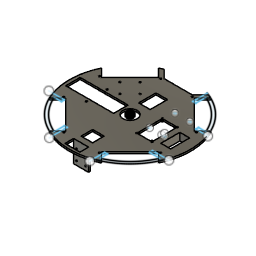
全国ディフェンス上面v3 v4 (Autodesk Fusion 360 design; units mm, degrees)
Autodesk Fusion 360 part; units mm, degrees
note: some values were not read from the file. Set by a fixed rule: which sketch regions a step uses.
sketch "スケッチ1" plane through (0, 0, 0) normal (0, 0, 1) x (1, 0, 0)
sketch "スケッチ2" plane through (0, 0, 0) normal (0, 0, 1) x (1, 0, 0)
  line L0 (105, 0) -> (105, 35)
  line L1 (105, 35) -> (98.9949, 35)
  line L2 (98.9949, 35) -> (78.9949, 35)
  line L3 (78.9949, 35) -> (105, 35)
  line L4 (105, 35) -> (105, -35)
  line L5 (105, -35) -> (78.9949, -35)
  line L6 (78.9949, -35) -> (78.9949, 35)
  line L7 (0, 105) -> (35, 105)
  line L8 (35, 105) -> (-35, 105)
  line L9 (-35, 105) -> (-35, 78.995)
  line L10 (-35, 78.995) -> (35, 78.995)
  line L11 (35, 78.995) -> (35, 105)
  line L12 (-105, 0) -> (-105, -35)
  line L13 (-105, -35) -> (-78.995, -35)
  line L14 (-78.995, -35) -> (-78.995, 34.9927)
  line L15 (-78.995, 34.9927) -> (-105, 34.9927)
  line L16 (-105, 34.9927) -> (-105, -35)
  line L17 (0, -105) -> (35, -105)
  line L18 (35, -105) -> (-35, -105)
  line L19 (-35, -105) -> (-35, -78.995)
  line L20 (-35, -78.995) -> (35, -78.995)
  line L21 (35, -78.995) -> (35, -105)
  arc A0 (-98.9949, -35) -> (-35, -98.9949) centre (0, 0) ccw
  arc A1 (35, -98.9949) -> (98.9949, -35) centre (0, 0) ccw
  arc A2 (98.9949, 35) -> (35, 98.9949) centre (0, 0) ccw
  arc A3 (-35, 98.9949) -> (-98.9975, 34.9927) centre (0, 0) ccw
  line L22 (-35, 98.9949) -> (-42, 98.9949)
  line L23 (-42, 98.9949) -> (-42, 96.2341)
  line L24 (-42, 96.2341) -> (-42, 76.2341)
  line L25 (-98.9975, 34.9927) -> (-98.9975, 42)
  line L26 (-98.9975, 42) -> (-96.2341, 42)
  line L27 (-96.2341, 42) -> (-76.2341, 42)
  line L28 (-76.2341, 42) -> (-42, 76.2341)
  dimension "d2" = 35
  dimension "d3" = 20
  dimension "d4" = 70
  dimension "d5" = 26.005
  dimension "d6" = 26.005
  dimension "d7" = 70
  dimension "d8" = 26.005
  dimension "d9" = 20
  dimension "d10" = 20
  constraint vertical L0
  constraint perpendicular L0 L1
  constraint perpendicular L0 L2
  constraint horizontal L3
  constraint vertical L4
  constraint horizontal L5
  constraint vertical L6
  constraint horizontal L7
  constraint horizontal L8
  constraint vertical L9
  constraint horizontal L10
  constraint vertical L11
  constraint vertical L12
  constraint horizontal L13
  constraint vertical L14
  constraint horizontal L15
  constraint vertical L16
  constraint horizontal L17
  constraint horizontal L18
  constraint vertical L19
  constraint horizontal L20
  constraint vertical L21
  constraint coincident L13 A0.start
  constraint coincident L19 A0.end
  constraint coincident L5 A1.end
  constraint coincident L21 A1.start
  constraint coincident L11 A2.end
  constraint coincident A0.centre A1.centre
  constraint coincident L15 A3.end
  constraint coincident L9 A3.start
  constraint perpendicular L9 L22
  constraint coincident A3 L23.end
  constraint perpendicular L22 L23
  constraint perpendicular L22 L24
  constraint perpendicular L15 L25
  constraint coincident A3 L26.end
  constraint perpendicular L25 L26
  constraint parallel L26 L27
  measures "d2" distance of L0.start L0.end
  measures "d3" distance of L1.end L2.end
  measures "d4" distance of L7.end L8.end
  measures "d5" distance of L7.end L10.end
  measures "d6" distance of L12.end L13.end
  measures "d7" distance of L17.end L18.end
  measures "d8" distance of L17.end L20.end
  measures "d9" distance of L23.end L24.end
  measures "d10" distance of L26.end L27.end
sketch "スケッチ3" plane through (0, 0, 0) normal (0, 0, 1) x (1, 0, 0)
  line L0 (-79, 35) -> (-74, 35)
  line L1 (-76.5, 35) -> (-76.5, 37.5)
  line L2 (-35, 79) -> (-35, 74)
  line L3 (-35, 74) -> (-35, 75)
  line L4 (-35, 76.5) -> (-37.5, 76.5)
  circle A0 centre (-37.5, 76.5) radius 1.5
  circle A1 centre (-76.5, 37.5) radius 1.5
  dimension "d11" = 3
  dimension "d12" = 3
  constraint horizontal L0
  constraint midpoint L0 L1.start
  constraint perpendicular L0 L1
  constraint vertical L2
  constraint coincident L2 L3.end
  constraint midpoint L2 L4.start
  constraint perpendicular L2 L4
  constraint coincident L4.end A0.centre
  constraint coincident L1.end A1.centre
  measures "d11" diameter of A0
  measures "d12" diameter of A1
extrude "押し出し1" add sketch "スケッチ2" along normal blind 3 contours L2 L3 L5 L6 L9 L10 L11 L13 L14 L15 L19 L20 L21 A0 A1 A2 A3 L24 L27 L28
extrude "押し出し2" cut sketch "スケッチ3" along normal blind 3
sketch "スケッチ4" plane through (0, 0, 0) normal (0, 0, 1) x (1, 0, 0)
sketch "スケッチ5" plane through (0, 0, 3) normal (0, 0, 1) x (-1, 0, 0)
  circle A0 centre (76.5, -37.5) radius 1.5
  circle A1 centre (37.5, -76.5) radius 1.5
  arc A2 (96.2341, -42) -> (98.9975, -34.9927) centre (0, 0) ccw
  line L0 (98.9975, -34.9927) -> (78.995, -34.9927)
  line L1 (78.995, -34.9927) -> (78.995, 35)
  line L2 (78.995, 35) -> (98.9949, 35)
  arc A3 (98.9949, 35) -> (35, 98.9949) centre (0, 0) ccw
  line L3 (35, 98.9949) -> (35, 78.995)
  line L4 (35, 78.995) -> (-35, 78.995)
  line L5 (-35, 78.995) -> (-35, 98.9949)
  arc A4 (-35, 98.9949) -> (-98.9949, 35) centre (0, 0) ccw
  line L6 (-98.9949, 35) -> (-78.9949, 35)
  line L7 (-78.9949, 35) -> (-78.9949, -35)
  line L8 (-78.9949, -35) -> (-98.9949, -35)
  arc A5 (-98.9949, -35) -> (-35, -98.9949) centre (0, 0) ccw
  line L9 (-35, -98.9949) -> (-35, -78.995)
  line L10 (-35, -78.995) -> (35, -78.995)
  line L11 (35, -78.995) -> (35, -98.9949)
  arc A6 (35, -98.9949) -> (42, -96.2341) centre (0, 0) ccw
  line L12 (42, -96.2341) -> (42, -76.2341)
  line L13 (42, -76.2341) -> (76.2341, -42)
  line L14 (76.2341, -42) -> (96.2341, -42)
  line L15 (78.995, -34.9927) -> (78.995, -40)
  line L16 (78.995, -40) -> (74, -40)
  line L17 (35, -78.995) -> (40, -78.995)
  line L18 (40, -78.995) -> (40, -74)
  line L19 (40, -74) -> (74, -40)
  constraint coincident L0.end L1.start
  constraint perpendicular L0 L15
  constraint perpendicular L15 L16
  constraint coincident L10.end L11.start
  constraint perpendicular L11 L17
  constraint perpendicular L10 L18
sketch "スケッチ6" plane through (0, 0, 3) normal (0, 0, 1) x (-1, 0, 0)
  line L0 (-35, -79) -> (-35, -74)
  line L1 (-35, -74) -> (-40, -74)
  arc A0 (-91.6515, -40) -> (-40, -91.6515) centre (0, 0) ccw
  line L2 (-79, -35) -> (-100, -35)
  line L3 (-79, -35) -> (-79, -40)
  arc A1 (-98.9949, -35) -> (-34.9984, -98.9955) centre (0, 0) ccw
  line L4 (-34.9984, -98.9955) -> (-35, -79)
  line L5 (-40, -74) -> (-40, -91.6515)
  line L6 (-91.6515, -40) -> (-79, -40)
  line L7 (-79, 35) -> (-74, 35)
  line L8 (-74, 35) -> (-74, 40)
  line L9 (-79, 35) -> (-102.5239, 35)
  line L10 (-35, 79) -> (-40, 79)
  line L11 (-35, 79) -> (-35, 105)
  arc A2 (-35, 98.9949) -> (-98.9949, 35) centre (0, 0) ccw
  arc A3 (-40, 91.6515) -> (-91.6515, 40) centre (0, 0) ccw
  line L12 (-40, 79) -> (-40, 91.6515)
  line L13 (-74, 40) -> (-91.6515, 40)
  line L14 (35, 79) -> (35, 74)
  line L15 (35, 74) -> (40, 74)
  line L16 (35, 79) -> (35, 105)
  line L17 (79, 35) -> (79, 40)
  line L18 (79, 35) -> (106, 35)
  arc A4 (98.9949, 35) -> (35, 98.9949) centre (0, 0) ccw
  arc A5 (91.6515, 40) -> (40, 91.6515) centre (0, 0) ccw
  line L19 (91.6515, 40) -> (79, 40)
  line L20 (40, 74) -> (40, 91.6515)
  dimension "d17" = 100
  dimension "d18" = 105
  dimension "d19" = 105
  dimension "d20" = 100
  dimension "d21" = 105
  dimension "d22" = 100
  constraint vertical L0
  constraint perpendicular L0 L1
  constraint coincident A0.centre A1.centre
  constraint perpendicular L2 L3
  constraint coincident L2 A1.start
  constraint perpendicular L1 L5
  constraint perpendicular L3 L6
  constraint horizontal L7
  constraint perpendicular L7 L8
  constraint parallel L7 L9
  constraint horizontal L10
  constraint perpendicular L10 L11
  constraint coincident L11 A2.start
  constraint coincident L9 A2.end
  constraint perpendicular L10 L12
  constraint perpendicular L8 L13
  constraint vertical L14
  constraint perpendicular L14 L15
  constraint parallel L14 L16
  constraint vertical L17
  constraint perpendicular L17 L18
  constraint coincident L18 A4.start
  constraint coincident L16 A4.end
  constraint perpendicular L17 L19
  constraint perpendicular L15 L20
  measures "d17" radius of A0
  measures "d18" radius of A1
  measures "d19" radius of A2
  measures "d20" radius of A3
  measures "d21" radius of A4
  measures "d22" radius of A5
sketch "スケッチ7" plane through (0, 0, 3) normal (0, 0, 1) x (-1, 0, 0)
  line L0 (79, 35) -> (74, 35)
  line L1 (76.5, 35) -> (76.5, 37.5)
  line L2 (37.5, 74) -> (37.5, 76.5)
  line L3 (-37.5, 79) -> (-37.5, 76.5)
  line L4 (-74, 37.5) -> (-76.5, 37.5)
  circle A0 centre (-76.5, -37.5) radius 1.5
  circle A1 centre (-37.5, -76.5) radius 1.5
  circle A2 centre (-76.5, 37.5) radius 1.5
  circle A3 centre (-37.5, 76.5) radius 1.5
  circle A4 centre (37.5, 76.5) radius 1.5
  circle A5 centre (76.5, 37.5) radius 1.5
  dimension "d23" = 2.5
  dimension "d24" = 3
  dimension "d25" = 3
  constraint horizontal L0
  constraint midpoint L0 L1.start
  constraint perpendicular L0 L1
  constraint vertical L2
  constraint vertical L3
  constraint horizontal L4
  constraint coincident L4.end A2.centre
  constraint coincident L3.end A3.centre
  constraint coincident L2.end A4.centre
  constraint coincident L1.end A5.centre
  measures "d23" distance of L1.start L1.end
  measures "d24" diameter of A2
  measures "d25" diameter of A5
extrude "押し出し3" cut sketch "スケッチ7" against normal blind 3
sketch "スケッチ8" plane through (0, 0, 3) normal (0, 0, 1) x (-1, 0, 0)
  line L0 (-68, 68) -> (-59.1612, 76.8388)
  line L1 (-68, 68) -> (-76.8388, 59.1612)
  line L2 (-76.8388, 59.1612) -> (-20.9774, 3.2997)
  line L3 (-20.9774, 3.2997) -> (-3.2997, 20.9774)
  line L4 (-3.2997, 20.9774) -> (-59.1612, 76.8388)
  line L5 (-76.8388, 59.1612) -> (-80.7279, 55.2721)
  line L6 (-80.7279, 55.2721) -> (-55.2721, 29.8162)
  line L7 (-55.2721, 29.8162) -> (-51.383, 33.7053)
  line L8 (-51.7365, 26.2807) -> (-47.8475, 30.1698)
  arc A0 (-55.2721, 29.8162) -> (-51.7365, 26.2807) centre (-53.5043, 28.0485) ccw
  circle A1 centre (-53.5043, 28.0485) radius 1.5
  line L9 (-53.5043, 28.0485) -> (-28.0485, 53.5043)
  circle A2 centre (-28.0485, 53.5043) radius 1.5
  dimension "d28" = 12.5
  dimension "d29" = 12.5
  dimension "d30" = 79
  dimension "d31" = 25
  dimension "d33" = 5.5
  dimension "d34" = 36
  dimension "d35" = 5
  dimension "d36" = 3
  dimension "d37" = 36
  dimension "d38" = 3
  constraint perpendicular L1 L2
  constraint perpendicular L2 L5
  constraint perpendicular L5 L6
  constraint coincident L2 L7.end
  constraint perpendicular L2 L7
  constraint coincident L2 L8.end
  constraint perpendicular L2 L8
  constraint concentric A0 A1
  constraint coincident A0.centre A1.centre
  constraint perpendicular L4 L9
  constraint coincident L9.end A2.centre
  measures "d28" distance of L0.start L0.end
  measures "d29" distance of L0.start L1.end
  measures "d30" distance of L1.end L2.end
  measures "d31" distance of L2.end L3.end
  measures "d33" distance of L1.end L5.end
  measures "d34" distance of L5.end L6.end
  measures "d35" distance of L6.end L8.start
  measures "d36" diameter of A1
  measures "d37" distance of A0.centre L9.end
  measures "d38" diameter of A2
extrude "押し出し4" cut sketch "スケッチ8" against normal blind 3 contours A1 | A2
sketch "スケッチ9" plane through (0, 0, 3) normal (0, 0, 1) x (-1, 0, 0)
  line L0 (-53.5, 28) -> (-81.4307, 55.9307)
  arc A0 (-55.2678, 29.7678) -> (-51.7322, 26.2322) centre (-53.5, 28) ccw
  line L1 (-55.2678, 29.7678) -> (-51.3787, 33.6569)
  line L2 (-81.4307, 55.9307) -> (-77.5416, 59.8198)
  line L3 (-77.5416, 59.8198) -> (-21.6802, 3.9584)
  line L4 (-21.6802, 3.9584) -> (-4.0025, 21.636)
  line L5 (-4.0025, 21.636) -> (-59.864, 77.4975)
  line L6 (-59.864, 77.4975) -> (-77.5416, 59.8198)
  dimension "d43" = 39.5
  dimension "d44" = 2.5
  dimension "d45" = 5.5
  dimension "d46" = 5.5
  dimension "d47" = 79
  dimension "d48" = 25
  dimension "d49" = 79
  constraint coincident L0.start A0.centre
  constraint perpendicular L0 L1
  constraint perpendicular L0 L2
  constraint perpendicular L1 L3
  constraint perpendicular L4 L5
  constraint perpendicular L3 L6
  measures "d43" distance of L0.start L0.end
  measures "d44" radius of A0
  measures "d45" distance of A0.start L1.end
  measures "d46" distance of L0.end L2.end
  measures "d47" distance of L2.end L3.end
  measures "d48" distance of L3.end L4.end
  measures "d49" distance of L4.end L5.end
extrude "押し出し5" cut sketch "スケッチ9" against normal blind 90 contours L3 L4 L5 L6
sketch "スケッチ10" plane through (0, 0, 3) normal (0, 0, 1) x (-1, 0, 0)
sketch "スケッチ11" plane through (0, 0, 0) normal (0, 0, 1) x (1, 0, 0)
sketch "スケッチ12" plane through (0, 0, 0) normal (0, 0, 1) x (1, 0, 0)
sketch "スケッチ13" plane through (0, 0, 0) normal (0, 0, 1) x (1, 0, 0)
sketch "スケッチ14" plane through (0, 0, 3) normal (0, 0, 1) x (-1, 0, 0)
  circle A0 centre (76.5, 37.5) radius 1.5
  circle A1 centre (37.5, 76.5) radius 1.5
  circle A2 centre (-37.5, 76.5) radius 1.5
  circle A3 centre (-76.5, 37.5) radius 1.5
  circle A4 centre (-76.5, -37.5) radius 1.5
  circle A5 centre (-37.5, -76.5) radius 1.5
  dimension "d71" = 3
  measures "d71" diameter of A0
extrude "押し出し6" add sketch "スケッチ14" against normal blind 3
sketch "スケッチ15" plane through (0, 0, 3) normal (0, 0, 1) x (-1, 0, 0)
extrude "押し出し7" add sketch "スケッチ5" along normal blind 3
move_face "面をオフセット1" offset -3 1 faces at (-50.128, -6.7155, 0)
sketch "スケッチ16" plane through (0, 0, 0) normal (0, 0, 1) x (1, 0, 0)
move_body "移動1" bodies 1 to x (0.707107, -0.707107, 0) y (0.707107, 0.707107, 0) z (0, 0, 1) at (-0.0004, -0.0009, -3)
sketch "スケッチ17" plane through (0, 0, 0) normal (0, 0, 1) x (1, 0, 0)
  line L0 (0, 0) -> (-16, 0)
  line L1 (-16, 0) -> (-16, 12.5)
  line L2 (-16, 12.5) -> (-99.104, 12.5)
  line L3 (-99.104, 12.5) -> (-99.104, -12.5)
  line L4 (-99.104, -12.5) -> (-16, -12.5)
  line L5 (-16, -12.5) -> (-16, 12.5)
  circle A0 centre (0, 0) radius 12.5
  line L6 (-57.552, 12.5) -> (-57.552, 0)
  line L7 (-57.552, 0) -> (-57.552, 18)
  line L8 (-57.552, 18) -> (-99.0603, 18)
  line L9 (-57.552, 18) -> (-57.552, -18)
  circle A1 centre (-57.552, 18) radius 1.5
  circle A2 centre (-57.552, -18) radius 1.5
  dimension "d77" = 16
  dimension "d78" = 12.5
  dimension "d79" = 83.104
  dimension "d80" = 25
  dimension "d81" = 25
  dimension "d82" = 18
  dimension "d84" = 3
  dimension "d85" = 3
  constraint coincident L0.start A0.centre
  constraint horizontal L0
  constraint perpendicular L0 L1
  constraint horizontal L2
  constraint vertical L3
  constraint horizontal L4
  constraint vertical L5
  constraint midpoint L2 L6.start
  constraint perpendicular L2 L6
  constraint perpendicular L2 L7
  constraint perpendicular L7 L8
  constraint perpendicular L4 L9
  constraint coincident L7.end L8.start
  constraint coincident L9.end A2.centre
  measures "d77" distance of L0.start L0.end
  measures "d78" distance of L0.end L1.end
  measures "d79" distance of L1.end L2.end
  measures "d80" distance of L1.end L4.end
  measures "d81" diameter of A0
  measures "d82" distance of L6.end L7.end
  measures "d84" diameter of A1
  measures "d85" diameter of A2
extrude "押し出し8" cut sketch "スケッチ17" along normal blind 3
sketch "スケッチ18" plane through (0, 0, 0) normal (0, 0, 1) x (1, 0, 0)
  circle A0 centre (60, 44) radius 1.5
  circle A1 centre (34, 44) radius 1.5
  circle A2 centre (60, 0) radius 1.5
  circle A3 centre (34, 0) radius 1.5
  line L0 (55, 0) -> (55, 5)
  dimension "d88" = 26
  dimension "d89" = 44
  dimension "d90" = 3
  dimension "d91" = 3
  dimension "d92" = 3
  dimension "d93" = 3
  measures "d88" distance of A2.centre A3.centre
  measures "d89" distance of A0.centre A2.centre
  measures "d90" diameter of A0
  measures "d91" diameter of A1
  measures "d92" diameter of A2
  measures "d93" diameter of A3
sketch "スケッチ19" plane through (0, 0, 0) normal (0, 0, -1) x (1, 0, 0)
  line L0 (-99.104, 12.5) -> (-16, 12.5)
  line L1 (-16, 12.5) -> (-16, -12.5)
  line L2 (-16, -12.5) -> (-99.104, -12.5)
  line L3 (-99.104, -12.5) -> (-99.104, 12.5)
  circle A0 centre (-57.552, -18) radius 1.5
  circle A1 centre (0, 0) radius 12.5
  circle A2 centre (-57.552, 18) radius 1.5
  circle A3 centre (-27.5775, -80.6093) radius 1.5
  circle A4 centre (27.5768, -80.6093) radius 1.5
  arc A5 (-45.2586, -94.7445) -> (-38.3497, -97.7454) centre (-0.0004, 0.0009) ccw
  line L4 (-38.3497, -97.7454) -> (-24.2075, -83.6032)
  line L5 (-24.2075, -83.6032) -> (24.2068, -83.6032)
  line L6 (24.2068, -83.6032) -> (38.3489, -97.7454)
  arc A6 (38.3489, -97.7454) -> (45.2509, -94.7478) centre (-0.0004, 0.0009) ccw
  line L7 (45.2509, -94.7478) -> (31.1088, -80.6057)
  line L8 (31.1088, -80.6057) -> (80.6063, -31.1083)
  line L9 (80.6063, -31.1083) -> (94.7484, -45.2504)
  arc A7 (94.7484, -45.2504) -> (94.7484, 45.2522) centre (-0.0004, 0.0009) ccw
  line L10 (94.7484, 45.2522) -> (80.6062, 31.11)
  line L11 (80.6062, 31.11) -> (31.1088, 80.6075)
  line L12 (31.1088, 80.6075) -> (45.2509, 94.7496)
  arc A8 (45.2509, 94.7496) -> (-45.2516, 94.7496) centre (-0.0004, 0.0009) ccw
  line L13 (-45.2516, 94.7496) -> (-31.1095, 80.6075)
  line L14 (-31.1095, 80.6075) -> (-80.607, 31.1101)
  line L15 (-80.607, 31.1101) -> (-94.7491, 45.2522)
  arc A9 (-94.7491, 45.2522) -> (-94.7491, -45.2504) centre (-0.0004, 0.0009) ccw
  line L16 (-94.7491, -45.2504) -> (-80.607, -31.1083)
  line L17 (-80.607, -31.1083) -> (-31.1147, -80.6006)
  line L18 (-31.1147, -80.6006) -> (-45.2586, -94.7445)
  line L19 (57.5, -22) -> (57.5, -19.5)
  line L20 (57.5, -19.5) -> (60, -19.5)
  line L21 (60, -19.5) -> (60, -22)
  line L22 (36.5, -22) -> (36.5, -19.5)
  line L23 (36.5, -19.5) -> (34, -19.5)
  line L24 (36.5, 22) -> (36.5, 19.5)
  line L25 (36.5, 19.5) -> (34, 19.5)
  line L26 (57.5, 22) -> (57.5, 19.5)
  line L27 (57.5, 19.5) -> (60, 19.5)
  line L28 (60, 19.5) -> (60, -19.5)
  line L29 (57.5, -22) -> (36.5, -22)
  line L30 (34, -19.5) -> (34, 19.5)
  line L31 (36.5, 22) -> (57.5, 22)
  circle A10 centre (60, -22) radius 1.5
  circle A11 centre (34, -22) radius 1.5
  circle A12 centre (60, 22) radius 1.5
  circle A13 centre (34, 22) radius 1.5
  dimension "d94" = 3
  dimension "d95" = 3
  dimension "d96" = 3
  dimension "d97" = 3
  constraint vertical L19
  constraint horizontal L20
  constraint vertical L21
  constraint vertical L22
  constraint horizontal L23
  constraint vertical L24
  constraint horizontal L25
  constraint vertical L26
  constraint horizontal L27
  constraint perpendicular L27 L28
  constraint perpendicular L22 L29
  constraint perpendicular L25 L30
  constraint perpendicular L26 L31
  constraint coincident L21.end A10.centre
  measures "d94" diameter of A10
  measures "d95" diameter of A11
  measures "d96" diameter of A12
  measures "d97" diameter of A13
extrude "押し出し9" cut sketch "スケッチ19" against normal blind 3 contours L19 L20 L22 L23 L24 L25 L26 L27 L28 L29 L30 L31 | A10 | A11 | A12 | A13
sketch "スケッチ20" plane through (0, 0, 0) normal (0, 0, 1) x (1, 0, 0)
  line L0 (0, 0) -> (70, 0)
  line L1 (70, 0) -> (70, 16.5)
  line L2 (70, 16.5) -> (87, 16.5)
  line L3 (87, 16.5) -> (87, -16.5)
  line L4 (87, -16.5) -> (70, -16.5)
  line L5 (70, -16.5) -> (70, 16.5)
  dimension "d100" = 16.5
  dimension "d101" = 17
  dimension "d102" = 33
  constraint coincident L0.start origin
  constraint horizontal L0
  constraint perpendicular L0 L1
  constraint horizontal L2
  constraint vertical L3
  constraint horizontal L4
  constraint vertical L5
  measures "d100" distance of L0.end L1.end
  measures "d101" distance of L1.end L2.end
  measures "d102" distance of L1.end L4.end
extrude "押し出し10" cut sketch "スケッチ20" along normal blind 3
sketch "スケッチ21" plane through (0, 0, 0) normal (0, 0, 1) x (1, 0, 0)
  circle A0 centre (0, 0) radius 102
  line L0 (12, -100) -> (-13, -100)
  line L1 (-13, -100) -> (-13, -90)
  line L2 (-13, -90) -> (12, -90)
  line L3 (0, -90) -> (13, -90)
  line L4 (13, -90) -> (13, -100)
  line L5 (13, -100) -> (12, -100)
  dimension "d105" = 204
  constraint coincident A0.centre origin
  constraint horizontal L0
  constraint vertical L1
  constraint horizontal L2
  constraint coincident L2 L3.start
  constraint perpendicular L2 L4
  measures "d105" diameter of A0
extrude "押し出し11" cut sketch "スケッチ21" along normal blind 3 contours L0 L1 L2 L3 L4 L5
sketch "スケッチ22" plane through (0, 0, 0) normal (0, 0, 1) x (1, 0, 0)
  line L0 (13, -90) -> (-13, -90)
  line L1 (-13, -90) -> (-13, -87)
  line L2 (-13, -87) -> (13, -87)
  line L3 (13, -87) -> (13, -90)
  constraint horizontal L0
  constraint vertical L1
  constraint horizontal L2
  constraint vertical L3
extrude "押し出し12" add sketch "スケッチ22" against normal blind 35
sketch "スケッチ23" plane through (0, 0, 0) normal (0, 1, 0) x (1, 0, 0)
  line L0 (0, 0) -> (0, 28)
  line L1 (0, 28) -> (-8, 28)
  line L2 (0, 28) -> (8, 28)
  circle A0 centre (8, 28) radius 1.5
  circle A1 centre (-8, 28) radius 1.5
  dimension "d110" = 28
  dimension "d111" = 8
  dimension "d112" = 8
  dimension "d113" = 3
  dimension "d114" = 3
  constraint coincident L0.start origin
  constraint vertical L0
  constraint perpendicular L0 L1
  constraint perpendicular L0 L2
  constraint coincident L2.end A0.centre
  constraint coincident L1.end A1.centre
  measures "d110" distance of L0.start L0.end
  measures "d111" distance of L0.end L1.end
  measures "d112" distance of L0.end L2.end
  measures "d113" diameter of A0
  measures "d114" diameter of A1
extrude "押し出し13" cut sketch "スケッチ23" against normal blind 1000
sketch "スケッチ24" plane through (0, 0, 0) normal (0, 0, 1) x (1, 0, 0)
  line L0 (70, 0) -> (70, 18.5)
  line L1 (70, 18.5) -> (68, 18.5)
  line L2 (68, 18.5) -> (89, 18.5)
  line L3 (89, 18.5) -> (89, -18.5)
  line L4 (89, -18.5) -> (68, -18.5)
  line L5 (68, -18.5) -> (68, 18.5)
  line L6 (70, 0) -> (70, 16.5)
  line L7 (70, 16.5) -> (87, 16.5)
  line L8 (87, 16.5) -> (87, -16.5)
  line L9 (87, -16.5) -> (70, -16.5)
  line L10 (70, -16.5) -> (70, 16.5)
  dimension "d117" = 18.5
  dimension "d118" = 16.5
  dimension "d119" = 17
  dimension "d120" = 33
  constraint vertical L0
  constraint perpendicular L0 L1
  constraint horizontal L2
  constraint vertical L3
  constraint horizontal L4
  constraint vertical L5
  constraint parallel L0 L6
  constraint horizontal L7
  constraint vertical L8
  constraint horizontal L9
  constraint vertical L10
  measures "d117" distance of L0.start L0.end
  measures "d118" distance of L0.start L6.end
  measures "d119" distance of L6.end L7.end
  measures "d120" distance of L6.end L9.end
extrude "押し出し14" add sketch "スケッチ24" against normal blind 10
move_body "移動2" bodies 1 to x (0.707107, 0.707107, 0) y (-0.707107, 0.707107, 0) z (0, 0, 1) at (0, 0, 0)
sketch "スケッチ25" plane through (0, 0, 0) normal (0, 0, 1) x (1, 0, 0)
  line L0 (-78.995, 0) -> (-68.995, 0)
  circle A0 centre (-43.995, 12.5) radius 1.5
  circle A1 centre (-68.995, 12.5) radius 1.5
  circle A2 centre (-43.995, -12.5) radius 1.5
  circle A3 centre (-68.995, -12.5) radius 1.5
  dimension "d123" = 10
  dimension "d124" = 12.5
  dimension "d125" = 25
  dimension "d126" = 25
  dimension "d127" = 3
  dimension "d128" = 3
  dimension "d129" = 3
  dimension "d130" = 3
  constraint horizontal L0
  measures "d123" distance of L0.start L0.end
  measures "d124" distance of L0.end A3.centre
  measures "d125" distance of A2.centre A3.centre
  measures "d126" distance of A1.centre A3.centre
  measures "d127" diameter of A0
  measures "d128" diameter of A1
  measures "d129" diameter of A2
  measures "d130" diameter of A3
extrude "押し出し15" cut sketch "スケッチ25" along normal blind 3
sketch "スケッチ26" plane through (0, 0, 0) normal (0, 0, 1) x (1, 0, 0)
  line L0 (35, 79) -> (40, 79)
  line L1 (37.5, 79) -> (37.5, 81.5)
  line L2 (79, 37.5) -> (81.5, 37.5)
  line L3 (79, -37.5) -> (81.5, -37.5)
  line L4 (37.5, -79) -> (37.5, -81.5)
  line L5 (-37.5, -79) -> (-37.5, -81.5)
  line L6 (-79, -37.5) -> (-81.5, -37.5)
  circle A0 centre (37.5, 81.5) radius 1.5
  circle A1 centre (81.5, 37.5) radius 1.5
  circle A2 centre (37.5, -81.5) radius 1.5
  circle A3 centre (81.5, -37.5) radius 1.5
  circle A4 centre (-37.5, -81.5) radius 1.5
  circle A5 centre (-81.5, -37.5) radius 1.5
  dimension "d133" = 3
  dimension "d134" = 3
  dimension "d135" = 3
  dimension "d136" = 3
  dimension "d137" = 3
  dimension "d138" = 3
  constraint horizontal L0
  constraint midpoint L0 L1.start
  constraint perpendicular L0 L1
  constraint horizontal L2
  constraint horizontal L3
  constraint vertical L4
  constraint vertical L5
  constraint horizontal L6
  constraint coincident L1.end A0.centre
  constraint coincident L2.end A1.centre
  constraint coincident L4.end A2.centre
  constraint coincident L3.end A3.centre
  constraint coincident L5.end A4.centre
  constraint coincident L6.end A5.centre
  measures "d133" diameter of A0
  measures "d134" diameter of A1
  measures "d135" diameter of A2
  measures "d136" diameter of A3
  measures "d137" diameter of A4
  measures "d138" diameter of A5
extrude "押し出し16" cut sketch "スケッチ26" along normal blind 3
sketch "スケッチ27" plane through (0, 0, 0) normal (0, 0, 1) x (1, 0, 0)
move_body "移動3" bodies 1 to x (0.707107, -0.707107, 0) y (0.707107, 0.707107, 0) z (0, 0, 1) at (0, 0, 0)
sketch "スケッチ28" plane through (0, 0, 0) normal (0, 0, 1) x (1, 0, 0)
  line L0 (10, -80) -> (-10, -80)
  line L1 (-10, -80) -> (-10, -60)
  line L2 (-10, -60) -> (10, -60)
  line L3 (10, -60) -> (10, -80)
  constraint horizontal L0
  constraint vertical L1
  constraint horizontal L2
  constraint vertical L3
extrude "押し出し17" cut sketch "スケッチ28" along normal blind 45
sketch "スケッチ29" plane through (0, 0, 0) normal (0, 0, 1) x (1, 0, 0)
  line L0 (10, 25) -> (-10, 25)
  line L1 (-10, 25) -> (-10, 55)
  line L2 (-10, 55) -> (10, 55)
  line L3 (10, 55) -> (10, 25)
  constraint horizontal L0
  constraint vertical L1
  constraint horizontal L2
  constraint vertical L3
extrude "押し出し18" cut sketch "スケッチ29" along normal blind 3
sketch "スケッチ30" plane through (0, 0, 0) normal (0, 0, 1) x (1, 0, 0)
  line L0 (-10, -60) -> (10, -60)
  line L1 (10, -60) -> (10, -80)
  line L2 (10, -80) -> (-10, -80)
  line L3 (-10, -80) -> (-10, -60)
  constraint horizontal L0
  constraint vertical L1
  constraint horizontal L2
  constraint vertical L3
extrude "押し出し19" add sketch "スケッチ30" along normal blind 3
extrude "押し出し20" add 1 faces at (2.484, -87, -8.8679) along direction (0, 1, 0) blind 5
extrude "押し出し21" cut 1 faces at (2.484, -90, -8.8679) along direction (0, 1, 0) blind 5
sketch "スケッチ31" plane through (0, 0, 0) normal (0, 1, 0) x (1, 0, 0)
  line L0 (0, 0) -> (0, 10)
  line L1 (0, 10) -> (-8, 10)
  line L2 (0, 10) -> (8, 10)
  circle A0 centre (8, 10) radius 1.5
  circle A1 centre (-8, 10) radius 1.5
  dimension "d151" = 3
  dimension "d152" = 3
  constraint coincident L0.start origin
  constraint vertical L0
  constraint perpendicular L0 L1
  constraint perpendicular L0 L2
  constraint coincident L2.end A0.centre
  constraint coincident L1.end A1.centre
  measures "d151" diameter of A0
  measures "d152" diameter of A1
extrude "押し出し22" cut sketch "スケッチ31" against normal blind 900
sketch "スケッチ32" plane through (0, 0, 0) normal (0, 0, 1) x (1, 0, 0)
  line L0 (0, -75) -> (-10, -75)
  line L1 (-10, -75) -> (-10, -55)
  line L2 (-10, -55) -> (0, -55)
  line L3 (0, -75) -> (10, -75)
  line L4 (10, -75) -> (10, -55)
  line L5 (10, -55) -> (0, -55)
  constraint horizontal L0
  constraint vertical L1
  constraint horizontal L2
  constraint horizontal L3
  constraint vertical L4
  constraint horizontal L5
extrude "押し出し23" cut sketch "スケッチ32" along normal blind 5
sketch "スケッチ33" plane through (0, 0, 0) normal (0, 1, 0) x (1, 0, 0)
